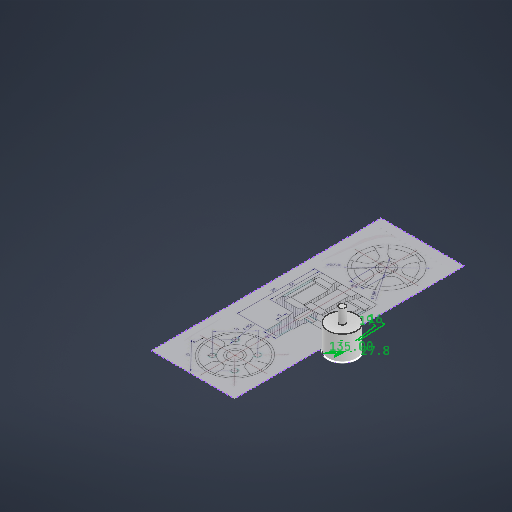
# Autodesk Inventor part: MOTOR
Saved by Autodesk Inventor 2025 (Build 290162010, 162A)
## iProperties
Created: 2025-05-21
Part Number: MOTOR
Material: Generic
Document SubType Name: Modeling
Designer: Jebediah Kerman
Density: 1 g/cm^3
Appearance: Default
Author: Jebediah Kerman
Autodesk Inventor part; units mm, degrees
ref_plane "YZ Plane" through (0, 0, 0) normal (1, 0, 0) x (0, 1, 0)
ref_plane "XZ Plane" through (0, 0, 0) normal (0, 1, 0) x (-1, 0, 0)
ref_plane "XY Plane" through (0, 0, 0) normal (0, 0, 1) x (1, 0, 0)
sketch "Sketch1" plane through (0, 0, 0) normal (0, 1, 0) x (-1, 0, 0)
  line L0 (93.6212, 93.2037) -> (93.6212, -131.4276) construction
  line L1 (93.6212, -131.4276) -> (12.1295, -131.4276) construction
  line L2 (12.1295, -131.4276) -> (12.1295, 93.2037) construction
  line L3 (12.1295, 93.2037) -> (93.6212, 93.2037) construction
  circle A0 centre (0, 0) radius 13.9
  circle A1 centre (0, 0) radius 8 construction
  circle A2 centre (0, 0) radius 9.5 construction
  line L4 (0, 0) -> (-9.8288, -9.8288) construction
  line L5 (0, 0) -> (13.9, 0) construction
  line L6 (0, 0) -> (9.8288, -9.8288) construction
  line L7 (0, 0) -> (9.8288, 9.8288) construction
  line L8 (0, 0) -> (-9.8288, 9.8288) construction
  point P0 (-6.7175, 6.7175)
  point P1 (-5.6569, -5.6569)
  point P2 (6.7175, -6.7175)
  point P3 (5.6569, 5.6569)
  dimension "d7" = 27.8
  dimension "d8" = 16
  dimension "d9" = 19
  dimension "d10" = 135
  constraints: 10 end point, 8 point on circle, 5 point on line, 3 centre point, 3 coincident, 1 equal length, 1 horizontal, 1 perpendicular, 2 other
  measures "d7" diameter of A0
  measures "d8" diameter of A1
  measures "d9" diameter of A2
  measures "d10" angle of L4 L5
extrude "Extrusion1" add sketch "Sketch1" along normal blind 24
hole "Hole1" at (6.7175, 0, 6.7175) at (5.6569, 0, -5.6569) at (-6.7175, 0, -6.7175) at (-5.6569, 0, 5.6569) direction (0, 1, 0) diameter 3 depth 4
sketch "Sketch2" plane through (0, 24, 0) normal (0, 1, 0) x (1, 0, 0)
  circle A0 centre (0, 0) radius 3
  dimension "d25" = 6
  constraints: 1 centre point, 1 coincident
  measures "d25" diameter of A0
extrude "Extrusion2" add sketch "Sketch2" along normal blind 14
body "Solid1"
